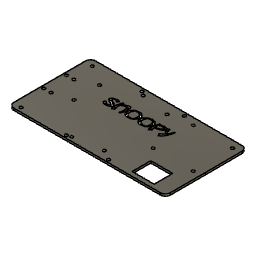
2nd and 3rd layer int round (Autodesk Fusion 360 design; units mm, degrees)
Autodesk Fusion 360 part; units mm, degrees
sketch "Sketch1" plane through (0, 0, 0) normal (0, 0, 1) x (1, 0, 0)
  line L0 (169.2354, 5) -> (169.2354, 40)
  line L1 (20, 82) -> (69, 82)
  line L2 (20, 0) -> (69, 0)
  circle A0 centre (20.1, 75.85) radius 1.5
  circle A1 centre (71.1, 75.85) radius 1.5
  circle A2 centre (20.1, 4.15) radius 1.5
  circle A3 centre (71.1, 4.15) radius 1.5
  circle A4 centre (99.5, 71.45) radius 1.5
  circle A5 centre (99.5, 8.55) radius 1.5
  line L3 (69, 82) -> (164.0857, 82)
  line L4 (69, 0) -> (164.2354, 0)
  arc A6 (169.0857, 77) -> (164.0857, 82) centre (164.0857, 77) ccw
  arc A7 (164.2354, 0) -> (169.2354, 5) centre (164.2354, 5) ccw
  circle A8 centre (67.0636, 78.781) radius 1.5
  circle A9 centre (109.5048, 78.781) radius 1.5
  circle A10 centre (109.5048, 2.781) radius 1.5
  circle A11 centre (67.0636, 2.781) radius 1.5
  line L5 (169.0857, 77) -> (169.2354, 40)
  line L6 (64.5023, 58.6453) -> (63.263, 56.9725)
  spline S0 degree 2 poles (63.263, 56.9725) (62.274, 58.1447) (60.6134, 58.1447) knots 0 0 0 1 1 1
  spline S1 degree 2 poles (60.6134, 58.1447) (60.2288, 58.1447) (59.9663, 58.0837) knots 0 0 0 1 1 1
  spline S2 degree 2 poles (59.9663, 58.0837) (60.4608, 58.5598) (60.9614, 59.036) knots 0 0 0 1 1 1
  spline S3 degree 2 poles (60.9614, 59.036) (61.4132, 59.3596) (62.1763, 59.3596) knots 0 0 0 1 1 1
  spline S4 degree 2 poles (62.1763, 59.3596) (63.4156, 59.3596) (64.5023, 58.6453) knots 0 0 0 1 1 1
  spline S5 degree 2 poles (65.3754, 52.1801) (65.3754, 50.8065) (63.9529, 49.8968) knots 0 0 0 1 1 1
  spline S6 degree 2 poles (63.9529, 49.8968) (62.7136, 49.0849) (61.2789, 49.0849) knots 0 0 0 1 1 1
  spline S7 degree 2 poles (61.2789, 49.0849) (61.9627, 49.4451) (62.4755, 49.9701) knots 0 0 0 1 1 1
  spline S8 degree 2 poles (62.4755, 49.9701) (63.1409, 50.6478) (63.1409, 51.2583) knots 0 0 0 1 1 1
  spline S9 degree 2 poles (63.1409, 51.2583) (63.1409, 52.0336) (61.4865, 52.7723) knots 0 0 0 1 1 1
  spline S10 degree 2 poles (61.4865, 52.7723) (59.9663, 53.4439) (58.4279, 54.1215) knots 0 0 0 1 1 1
  spline S11 degree 2 poles (58.4279, 54.1215) (56.7856, 55.0434) (56.7856, 56.2827) knots 0 0 0 1 1 1
  spline S12 degree 2 poles (56.7856, 56.2827) (56.7856, 57.1862) (58.0493, 58.0714) knots 0 0 0 1 1 1
  spline S13 degree 2 poles (58.0493, 58.0714) (59.075, 58.7979) (60.1495, 59.0849) knots 0 0 0 1 1 1
  spline S14 degree 2 poles (60.1495, 59.0849) (58.7758, 58.1569) (58.7758, 57.2839) knots 0 0 0 1 1 1
  spline S15 degree 2 poles (58.7758, 57.2839) (58.7758, 56.5696) (60.4913, 55.6478) knots 0 0 0 1 1 1
  spline S16 degree 2 poles (60.4913, 55.6478) (62.0786, 54.848) (63.6659, 54.0482) knots 0 0 0 1 1 1
  spline S17 degree 2 poles (63.6659, 54.0482) (65.3754, 53.0592) (65.3754, 52.1801) knots 0 0 0 1 1 1
  spline S18 degree 2 poles (61.8406, 50.0067) (61.3033, 49.671) (60.7783, 49.3169) knots 0 0 0 1 1 1
  spline S19 degree 2 poles (60.7783, 49.3169) (60.1373, 48.9445) (59.5878, 48.9445) knots 0 0 0 1 1 1
  spline S20 degree 2 poles (59.5878, 48.9445) (58.7636, 48.9445) (57.6647, 49.4573) knots 0 0 0 1 1 1
  spline S21 degree 2 poles (57.6647, 49.4573) (56.7368, 49.8968) (55.9248, 50.5073) knots 0 0 0 1 1 1
  line L7 (55.9248, 50.5073) -> (57.5487, 52.4304)
  spline S22 degree 2 poles (57.5487, 52.4304) (58.202, 51.3926) (59.2398, 50.721) knots 0 0 0 1 1 1
  spline S23 degree 2 poles (59.2398, 50.721) (60.3631, 49.9945) (61.5109, 49.9945) knots 0 0 0 1 1 1
  spline S24 degree 2 poles (61.5109, 49.9945) (61.6757, 49.9945) (61.8406, 50.0067) knots 0 0 0 1 1 1
  spline S25 degree 2 poles (76.0652, 56.0202) (76.0652, 52.7051) (74.4657, 48.9567) knots 0 0 0 1 1 1
  line L8 (74.4657, 48.9567) -> (73.5866, 49.268)
  spline S26 degree 2 poles (73.5866, 49.268) (74.252, 50.8065) (74.252, 52.7357) knots 0 0 0 1 1 1
  spline S27 degree 2 poles (74.252, 52.7357) (74.252, 55.1471) (73.4645, 57.1618) knots 0 0 0 1 1 1
  spline S28 degree 2 poles (73.4645, 57.1618) (72.9883, 57.3694) (72.39, 57.3694) knots 0 0 0 1 1 1
  spline S29 degree 2 poles (72.39, 57.3694) (70.5402, 57.3694) (68.3119, 55.9103) knots 0 0 0 1 1 1
  line L9 (68.3119, 55.9103) -> (68.3729, 56.9115)
  spline S30 degree 2 poles (68.3729, 56.9115) (69.6977, 58.0959) (71.4132, 58.8712) knots 0 0 0 1 1 1
  spline S31 degree 2 poles (71.4132, 58.8712) (73.2508, 59.7076) (74.8992, 59.7747) knots 0 0 0 1 1 1
  spline S32 degree 2 poles (74.8992, 59.7747) (76.0652, 58.4988) (76.0652, 56.0202) knots 0 0 0 1 1 1
  line L10 (68.8125, 49.5183) -> (66.4498, 48.5171)
  spline S33 degree 2 poles (66.4498, 48.5171) (66.0103, 50.0922) (66.0103, 52.406) knots 0 0 0 1 1 1
  spline S34 degree 2 poles (66.0103, 52.406) (66.0103, 56.3437) (67.622, 59.7076) knots 0 0 0 1 1 1
  line L11 (67.622, 59.7076) -> (68.2508, 59.207)
  spline S35 degree 2 poles (68.2508, 59.207) (67.6769, 57.3205) (67.6769, 54.8602) knots 0 0 0 1 1 1
  spline S36 degree 2 poles (67.6769, 54.8602) (67.6769, 51.8199) (68.8125, 49.5183) knots 0 0 0 1 1 1
  spline S37 degree 2 poles (89.191, 55.0189) (89.191, 53.2729) (87.9822, 51.6551) knots 0 0 0 1 1 1
  spline S38 degree 2 poles (87.9822, 51.6551) (86.8406, 50.1227) (85.18, 49.3962) knots 0 0 0 1 1 1
  spline S39 degree 2 poles (85.18, 49.3962) (87.042, 51.5818) (87.042, 54.0849) knots 0 0 0 1 1 1
  spline S40 degree 2 poles (87.042, 54.0849) (87.042, 55.8309) (85.7661, 57.2778) knots 0 0 0 1 1 1
  spline S41 degree 2 poles (85.7661, 57.2778) (84.4901, 58.7247) (82.7807, 58.7247) knots 0 0 0 1 1 1
  spline S42 degree 2 poles (82.7807, 58.7247) (82.2007, 58.7247) (81.6391, 58.5232) knots 0 0 0 1 1 1
  line L12 (81.6391, 58.5232) -> (82.8174, 59.6465)
  spline S43 degree 2 poles (82.8174, 59.6465) (83.3302, 59.7076) (83.8186, 59.7076) knots 0 0 0 1 1 1
  spline S44 degree 2 poles (83.8186, 59.7076) (85.9553, 59.7076) (87.5182, 58.45) knots 0 0 0 1 1 1
  spline S45 degree 2 poles (87.5182, 58.45) (89.191, 57.1069) (89.191, 55.0189) knots 0 0 0 1 1 1
  line L13 (84.9907, 50.5073) -> (84.1788, 49.207)
  spline S46 degree 2 poles (84.1788, 49.207) (83.1165, 48.9811) (82.1519, 48.9811) knots 0 0 0 1 1 1
  spline S47 degree 2 poles (82.1519, 48.9811) (79.8747, 48.9811) (78.4034, 50.196) knots 0 0 0 1 1 1
  spline S48 degree 2 poles (78.4034, 50.196) (76.8161, 51.4964) (76.8161, 53.7308) knots 0 0 0 1 1 1
  spline S49 degree 2 poles (76.8161, 53.7308) (76.8161, 55.5684) (78.2905, 57.3266) knots 0 0 0 1 1 1
  spline S50 degree 2 poles (78.2905, 57.3266) (79.7649, 59.0849) (81.578, 59.3352) knots 0 0 0 1 1 1
  spline S51 degree 2 poles (81.578, 59.3352) (80.3753, 58.395) (79.716, 57.1191) knots 0 0 0 1 1 1
  spline S52 degree 2 poles (79.716, 57.1191) (79.0261, 55.8065) (79.0261, 54.3352) knots 0 0 0 1 1 1
  spline S53 degree 2 poles (79.0261, 54.3352) (79.0261, 52.4426) (80.2197, 51.3071) knots 0 0 0 1 1 1
  spline S54 degree 2 poles (80.2197, 51.3071) (81.4132, 50.1716) (83.318, 50.1716) knots 0 0 0 1 1 1
  spline S55 degree 2 poles (83.318, 50.1716) (84.4047, 50.1716) (84.9907, 50.5073) knots 0 0 0 1 1 1
  spline S56 degree 2 poles (102.2679, 55.0189) (102.2679, 53.2729) (101.0591, 51.6551) knots 0 0 0 1 1 1
  spline S57 degree 2 poles (101.0591, 51.6551) (99.9175, 50.1227) (98.2569, 49.3962) knots 0 0 0 1 1 1
  spline S58 degree 2 poles (98.2569, 49.3962) (100.1189, 51.5818) (100.1189, 54.0849) knots 0 0 0 1 1 1
  spline S59 degree 2 poles (100.1189, 54.0849) (100.1189, 55.8309) (98.843, 57.2778) knots 0 0 0 1 1 1
  spline S60 degree 2 poles (98.843, 57.2778) (97.5671, 58.7247) (95.8576, 58.7247) knots 0 0 0 1 1 1
  spline S61 degree 2 poles (95.8576, 58.7247) (95.2777, 58.7247) (94.716, 58.5232) knots 0 0 0 1 1 1
  line L14 (94.716, 58.5232) -> (95.8943, 59.6465)
  spline S62 degree 2 poles (95.8943, 59.6465) (96.4071, 59.7076) (96.8955, 59.7076) knots 0 0 0 1 1 1
  spline S63 degree 2 poles (96.8955, 59.7076) (99.0323, 59.7076) (100.5951, 58.45) knots 0 0 0 1 1 1
  spline S64 degree 2 poles (100.5951, 58.45) (102.2679, 57.1069) (102.2679, 55.0189) knots 0 0 0 1 1 1
  line L15 (98.0677, 50.5073) -> (97.2557, 49.207)
  spline S65 degree 2 poles (97.2557, 49.207) (96.1934, 48.9811) (95.2288, 48.9811) knots 0 0 0 1 1 1
  spline S66 degree 2 poles (95.2288, 48.9811) (92.9517, 48.9811) (91.4804, 50.196) knots 0 0 0 1 1 1
  spline S67 degree 2 poles (91.4804, 50.196) (89.8931, 51.4964) (89.8931, 53.7308) knots 0 0 0 1 1 1
  spline S68 degree 2 poles (89.8931, 53.7308) (89.8931, 55.5684) (91.3674, 57.3266) knots 0 0 0 1 1 1
  spline S69 degree 2 poles (91.3674, 57.3266) (92.8418, 59.0849) (94.655, 59.3352) knots 0 0 0 1 1 1
  spline S70 degree 2 poles (94.655, 59.3352) (93.4523, 58.395) (92.7929, 57.1191) knots 0 0 0 1 1 1
  spline S71 degree 2 poles (92.7929, 57.1191) (92.1031, 55.8065) (92.1031, 54.3352) knots 0 0 0 1 1 1
  spline S72 degree 2 poles (92.1031, 54.3352) (92.1031, 52.4426) (93.2966, 51.3071) knots 0 0 0 1 1 1
  spline S73 degree 2 poles (93.2966, 51.3071) (94.4901, 50.1716) (96.3949, 50.1716) knots 0 0 0 1 1 1
  spline S74 degree 2 poles (96.3949, 50.1716) (97.4816, 50.1716) (98.0677, 50.5073) knots 0 0 0 1 1 1
  spline S75 degree 2 poles (111.981, 57.5953) (111.981, 55.6111) (109.5084, 54.5061) knots 0 0 0 1 1 1
  spline S76 degree 2 poles (109.5084, 54.5061) (107.6464, 53.6819) (105.3326, 53.6209) knots 0 0 0 1 1 1
  line L16 (105.3326, 53.6209) -> (105.2716, 54.5489)
  line L17 (105.2716, 54.5489) -> (105.4791, 54.5489)
  spline S77 degree 2 poles (105.4791, 54.5489) (107.0787, 54.5183) (108.2325, 55.196) knots 0 0 0 1 1 1
  spline S78 degree 2 poles (108.2325, 55.196) (109.6183, 55.9957) (109.6183, 57.5098) knots 0 0 0 1 1 1
  spline S79 degree 2 poles (109.6183, 57.5098) (109.6183, 57.9188) (108.8186, 58.2363) knots 0 0 0 1 1 1
  spline S80 degree 2 poles (108.8186, 58.2363) (108.1592, 58.511) (107.6586, 58.511) knots 0 0 0 1 1 1
  spline S81 degree 2 poles (107.6586, 58.511) (106.5536, 58.511) (105.3326, 57.7845) knots 0 0 0 1 1 1
  line L18 (105.3326, 57.7845) -> (105.2716, 58.5232)
  spline S82 degree 2 poles (105.2716, 58.5232) (105.8332, 59.036) (106.9443, 59.3596) knots 0 0 0 1 1 1
  spline S83 degree 2 poles (106.9443, 59.3596) (107.9334, 59.6465) (108.8064, 59.6465) knots 0 0 0 1 1 1
  spline S84 degree 2 poles (108.8064, 59.6465) (110.0091, 59.6465) (110.8699, 59.207) knots 0 0 0 1 1 1
  spline S85 degree 2 poles (110.8699, 59.207) (111.981, 58.6697) (111.981, 57.5953) knots 0 0 0 1 1 1
  line L19 (105.2716, 50.0067) -> (103.031, 48.7064)
  spline S86 degree 2 poles (103.031, 48.7064) (102.7441, 50.2326) (102.7441, 51.9054) knots 0 0 0 1 1 1
  spline S87 degree 2 poles (102.7441, 51.9054) (102.7441, 56.185) (104.1544, 59.7747) knots 0 0 0 1 1 1
  line L20 (104.1544, 59.7747) -> (104.8931, 59.1459)
  spline S88 degree 2 poles (104.8931, 59.1459) (104.368, 57.87) (104.368, 55.9347) knots 0 0 0 1 1 1
  spline S89 degree 2 poles (104.368, 55.9347) (104.368, 53.0226) (105.2716, 50.0067) knots 0 0 0 1 1 1
  line L21 (116.0347, 54.8724) -> (115.5585, 54.0849)
  spline S90 degree 2 poles (115.5585, 54.0849) (114.2215, 54.6221) (113.1348, 56.0568) knots 0 0 0 1 1 1
  spline S91 degree 2 poles (113.1348, 56.0568) (112.1458, 57.345) (111.694, 58.8834) knots 0 0 0 1 1 1
  line L22 (111.694, 58.8834) -> (114.0689, 59.9091)
  spline S92 degree 2 poles (114.0689, 59.9091) (114.2215, 58.4988) (114.6611, 57.2106) knots 0 0 0 1 1 1
  spline S93 degree 2 poles (114.6611, 57.2106) (115.2105, 55.5867) (116.0347, 54.8724) knots 0 0 0 1 1 1
  spline S94 degree 2 poles (119.3863, 59.4817) (119.136, 56.1972) (117.7197, 53.2485) knots 0 0 0 1 1 1
  spline S95 degree 2 poles (117.7197, 53.2485) (116.1202, 49.8968) (113.611, 48.395) knots 0 0 0 1 1 1
  line L23 (113.611, 48.395) -> (112.0725, 50.544)
  spline S96 degree 2 poles (112.0725, 50.544) (114.6367, 51.9481) (116.4071, 54.3474) knots 0 0 0 1 1 1
  spline S97 degree 2 poles (116.4071, 54.3474) (118.3363, 56.9481) (118.495, 59.671) knots 0 0 0 1 1 1
  line L24 (118.495, 59.671) -> (119.3863, 59.4817)
  circle A12 centre (40.1923, 63.0763) radius 1.5
  circle A13 centre (40.1923, 37.3733) radius 1.5
  circle A14 centre (122.0438, 75.0849) radius 1.5
  circle A15 centre (161.7205, 74.9646) radius 1.5
  circle A16 centre (121.8474, 35.1909) radius 1.5
  circle A17 centre (161.855, 35.2854) radius 1.5
  line L25 (131.6005, 23.0024) -> (153.6005, 23.0024)
  line L26 (153.6005, 23.0024) -> (153.6005, 4.3024)
  line L27 (153.6005, 4.3024) -> (131.6005, 4.3024)
  line L28 (131.6005, 4.3024) -> (131.6005, 23.0024)
  line L29 (25.2162, 82.0887) -> (62.2162, 82.0887)
  line L30 (62.2162, 82.0887) -> (62.2162, 32.0887)
  line L31 (62.2162, 32.0887) -> (25.2162, 32.0887)
  line L32 (25.2162, 32.0887) -> (25.2162, 82.0887)
  line L33 (20, 82) -> (17.1238, 82)
  line L34 (12.1238, 77) -> (12.1238, 5)
  line L35 (17.1238, 0) -> (20, 0)
  arc A18 (12.1238, 5) -> (17.1238, 0) centre (17.1238, 5) ccw
  arc A19 (17.1238, 82) -> (12.1238, 77) centre (17.1238, 77) ccw
  circle A20 centre (15, 55) radius 1.5
  circle A21 centre (22.4154, 55) radius 1.5
  circle A22 centre (15, 32.1656) radius 1.5
  circle A23 centre (22.4154, 32.1656) radius 1.5
  point P0 (15, 0)
  point P1 (15, 82)
  dimension "d20" = 54
  dimension "d21" = 54
  dimension "d22" = 3
  dimension "d23" = 3
  dimension "d24" = 6.15
  dimension "d25" = 6.15
  dimension "d27" = 51
  dimension "d56" = 82
  dimension "d58" = 3
  dimension "d76" = 71.7
  dimension "d77" = 71.7
  dimension "d78" = 5
  dimension "d79" = 5
  dimension "d83" = 3
  dimension "d84" = 3
  dimension "d85" = 3
  dimension "d86" = 3
  dimension "d94" = 76
  dimension "d95" = 76
  dimension "d98" = 3
  dimension "d99" = 3
  dimension "d102" = 3
  dimension "d103" = 3
  dimension "d104" = 3
  dimension "d105" = 3
  dimension "d106" = 22
  dimension "d107" = 18.7
  dimension "d112" = 37
  dimension "d113" = 50
  dimension "d116" = 5
  dimension "d117" = 3
  dimension "d118" = 3
  dimension "d119" = 3
  dimension "d120" = 3
  constraint coincident P1 L1
  constraint coincident P0 L2
  constraint parallel L1 L3
  constraint tangent L3 A6
  constraint tangent L0 A7
  constraint tangent L4 A7
  constraint horizontal L25
  constraint vertical L26
  constraint horizontal L27
  constraint vertical L28
  constraint horizontal L29
  constraint vertical L30
  constraint horizontal L31
  constraint vertical L32
  constraint horizontal L33
  constraint vertical L34
  constraint horizontal L35
  constraint tangent L34 A18
  constraint tangent L35 A18
  constraint tangent L34 A19
  constraint tangent L33 A19
  constraint equal A18 A19
  measures "d20" distance of P1 L1.end
  measures "d21" distance of P0 L2.end
  measures "d22" diameter of A0
  measures "d23" diameter of A1
  measures "d24" distance of L1 A0.centre
  measures "d25" distance of L1 A1.centre
  measures "d27" distance of A0.centre A1.centre
  measures "d56" distance of P0 P1
  measures "d58" diameter of A4
  measures "d76" distance of A0.centre A2.centre
  measures "d77" distance of A1.centre A3.centre
  measures "d78" radius of A6
  measures "d79" radius of A7
  measures "d83" diameter of A8
  measures "d84" diameter of A9
  measures "d85" diameter of A10
  measures "d86" diameter of A11
  measures "d94" distance of A9.centre A10.centre
  measures "d95" distance of A8.centre A11.centre
  measures "d98" diameter of A12
  measures "d99" diameter of A13
  measures "d102" diameter of A14
  measures "d103" diameter of A15
  measures "d104" diameter of A16
  measures "d105" diameter of A17
  measures "d106" distance of L25.start L25.end
  measures "d107" distance of L25.start L27.end
  measures "d112" distance of L29.start L29.end
  measures "d113" distance of L29.start L31.end
  measures "d116" radius of A18
  measures "d117" diameter of A20
  measures "d118" diameter of A21
  measures "d119" diameter of A22
  measures "d120" diameter of A23
extrude "Extrude6" add sketch "Sketch1" along normal blind 2 contours L0 L1 L2 L3 L4 A6 A7 L5 L6 S0 S4 S5 S6 S16 S17 L30 L31 L32 L33 L34 L35 A18 A19 | L1 S0 S1 S2 S3 S4 S6 S7 S9 S10 S11 S12 S13 S14 S15 S16 L30 L31 L32
